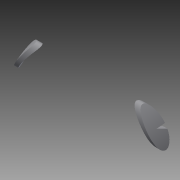
# Autodesk Inventor part: PacmanEye
Saved by Autodesk Inventor 2015 (Build 190159000, 159)
## iProperties
Created: 2015-04-11
Part Number: PacmanEye
Material: Generic
Document SubType Name: Modeling
Designer: tquinn
Density: 1 g/cm^3
Appearance: Default
Author: tquinn
Autodesk Inventor part; units mm, degrees
ref_plane "YZ Plane" through (0, 0, 0) normal (1, 0, 0) x (0, 1, 0)
ref_plane "XZ Plane" through (0, 0, 0) normal (0, 1, 0) x (-1, 0, 0)
ref_plane "XY Plane" through (0, 0, 0) normal (0, 0, 1) x (1, 0, 0)
sketch "Sketch1" plane through (0, 0, 0) normal (1, 0, 0) x (0, 1, 0)
  circle A0 centre (7.62, 4.445) radius 1.905
  line L0 (7.62, 4.445) -> (7.62, 2.54)
  line L1 (7.62, 4.445) -> (8.1131, 2.6049)
  line L2 (7.62, 4.445) -> (7.1269, 2.6049)
  ellipse E0 centre (7.62, 4.445) end of major axis (10.2659, 4.445) minor radius 1.2487
  line L3 (7.62, 4.445) -> (7.9519, 3.2062)
  line L4 (7.62, 4.445) -> (7.2881, 3.2062)
  point P0 (0, 0)
  dimension "d0" = 3.81
  dimension "d1" = 7.62
  dimension "d2" = 4.445
  dimension "d3" = 15
  dimension "d4" = 15
  constraints: 10 end point, 3 point on circle, 2 point on line, 1 centre point, 1 coincident, 1 vertical, 4 other
  measures "d0" diameter of A0
  measures "d1" horizontal distance of point (0, 0) L0.start
  measures "d2" vertical distance of point (0, 0) L0.start
  measures "d3" angle of L0 L1
  measures "d4" angle of L2 L0
extrude "Extrusion1" add sketch "Sketch1" along normal mid plane 50.8 contours E0 A0 | A0 E0 L1 L2 | A0 E0 picked at (5.4761, 4.4598) picked at (9.7253, 4.2127)
sketch "Sketch2" plane through (0, 0, 0) normal (1, 0, 0) x (0, 1, 0)
  arc A0 (-7.0261, 12.0881) -> (6.9439, 12.0881) centre (-0.0411, -0.0103) ccw
  circle A1 centre (-0.0411, -0.0103) radius 13.97
  circle A2 centre (-0.0411, -0.0103) radius 14.986
  line L0 (14.9449, -0.0103) -> (-15.0271, -0.0103)
  line L1 (14.9449, -0.0103) -> (13.9289, -0.0103)
  line L2 (-14.0111, -0.0103) -> (-15.0271, -0.0103)
  point P0 (0, 0)
  dimension "d7" = 1.016
  constraints: 6 end point, 6 point on circle, 3 centre point, 2 coincident, 2 point on line, 1 collinear, 1 concentric, 1 horizontal, 4 other
  measures "d7" radial gap between concentric circles of A0 A2
revolve "Revolution1" cut sketch "Sketch2" angle 360 about axis through (0, 14.9449, -0.0103) along (0, -1, 0) keep common part contours A0 L0 A2 A1
equation "\"d4\" = d3"
body "Solid1"
